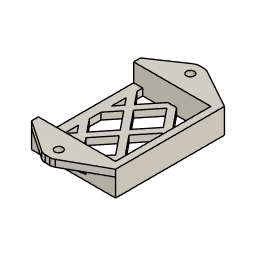
Top Motor Base_ (Autodesk Fusion 360 design; units mm, degrees)
Autodesk Fusion 360 part; units mm, degrees
sketch "Sketch1" plane through (0, 0, 0) normal (0, 0, 1) x (1, 0, 0)
  line L0 (0, 0) -> (-34, 0)
  line L1 (-34, 42) -> (0, 42)
  line L2 (0, 42) -> (0, 0)
  line L3 (-34, -3) -> (-34, 45)
  line L4 (3, -3) -> (-34, -3)
  line L5 (-34, 45) -> (3, 45)
  line L6 (3, 45) -> (3, -3)
  line L7 (-18, 55) -> (-16, 55)
  line L8 (-12, 51) -> (-12, 45)
  line L9 (-12, 45) -> (-22, 45)
  line L10 (-22, 45) -> (-22, 51)
  circle A0 centre (-17, 50) radius 1.75
  arc A1 (-18, 55) -> (-22, 51) centre (-18, 51) ccw
  arc A2 (-12, 51) -> (-16, 55) centre (-16, 51) ccw
  circle A3 centre (-17, -8) radius 1.75
  line L11 (-22, -3) -> (-22, -9)
  arc A4 (-22, -9) -> (-18, -13) centre (-18, -9) ccw
  line L12 (-18, -13) -> (-16, -13)
  arc A5 (-16, -13) -> (-12, -9) centre (-16, -9) ccw
  line L13 (-12, -9) -> (-12, -3)
  line L14 (3, 45) -> (-14.0543, 54.4949)
  line L15 (3, -3) -> (-14.0543, -12.4949)
  line L16 (-34, 45) -> (-20.2422, 54.3125)
  line L17 (-34, -3) -> (-20.2422, -12.3125)
  line L18 (-19.75, -9.5877) -> (-17, -11.1754)
  line L19 (-17, -11.1754) -> (-14.25, -9.5877)
  line L20 (-14.25, -9.5877) -> (-14.25, -6.4123)
  line L21 (-14.25, -6.4123) -> (-17, -4.8246)
  line L22 (-17, -4.8246) -> (-19.75, -6.4123)
  line L23 (-19.75, -6.4123) -> (-19.75, -9.5877)
  point P0 (-22, 55)
  point P1 (-12, 55)
  point P2 (-17, -8)
  dimension "d1" = 34
  dimension "d2" = 42
  dimension "d6" = 10
  dimension "d7" = 10
  dimension "d8" = 3.5
  dimension "d9" = 4
  dimension "d24" = 20
  dimension "d43" = 5
  dimension "d79" = 2.75
  constraint horizontal L0
  constraint vertical L3
  constraint horizontal L1
  constraint vertical L2
  constraint coincident L0.start L2.end
  constraint horizontal L7
  constraint vertical L8
  constraint horizontal L9
  constraint vertical L10
  constraint coincident P0 L7
  constraint coincident P0 L10
  constraint tangent L7 A1
  constraint tangent L10 A1
  constraint coincident P1 L7
  constraint coincident P1 L8
  constraint tangent L7 A2
  constraint tangent L8 A2
  constraint equal A1 A2
  constraint coincident A2 L14.end
  constraint tangent A2 L14
  constraint coincident A5 L15.end
  constraint tangent A5 L15
  constraint coincident L1.start L3
  constraint coincident L0.end L3
  constraint coincident A1 L16.end
  constraint tangent A1 L16
  constraint coincident A4 L17.end
  constraint tangent A4 L17
  constraint coincident P2 A3.centre
  constraint parallel L3 L23
  measures "d1" distance of L0.start L0.end
  measures "d2" distance of L0.start L1.end
  measures "d6" distance of P0 P1
  measures "d7" distance of P0 L9.end
  measures "d8" diameter of A0
  measures "d9" radius of A1
  measures "d24" distance of L6 A0.centre
  measures "d43" distance of L5 A0.centre
  measures "d79" distance of P2 L23
extrude "Extrude1" add sketch "Sketch1" along normal blind 11 contours L0 L1 L2 L3 L4 L5 L6 L9
extrude "Extrude2" add sketch "Sketch1" along normal blind 3 from surface at 8 contours L4 L11 A4 L17 | L4 L11 A4 L12 A5 L13 | L5 L10 A1 L16 | L4 A5 L13 L15 | L5 L7 L8 L9 L10 A1 A2 | L5 L8 A2 L14 | L18 L19 L20 L21 L22 L23
extrude "Extrude5" add sketch "Sketch1" along normal blind 3 contours L0 L1 L2 L3
ref_plane "WorkPlane3" through (0, 21, 0) normal (0, 1, 0) x (0, 0, 1)
sketch "Sketch5" plane through (0, 0, 3) normal (0, 0, 1) x (-1, 0, 0)
  line L0 (30, 0) -> (30, -42)
  line L1 (34, -42) -> (34, 0)
  line L2 (34, 0) -> (0, 0)
  line L3 (0, 0) -> (0, -42)
  line L4 (0, -42) -> (34, -42)
  line L5 (34, -42) -> (34, 0)
  line L6 (0, -21) -> (17, 0)
  line L7 (0, -42) -> (30, -4.9412)
  line L8 (17, -42) -> (30, -25.9412)
  line L9 (17, -42) -> (0, -21)
  line L10 (0, 0) -> (30, -37.0588)
  line L11 (30, -16.0588) -> (17, 0)
  line L12 (18.1659, -41.0562) -> (1.1659, -20.0562)
  line L13 (15.0701, -42) -> (0, -23.384)
  line L14 (1.9299, -42) -> (30, -7.3252)
  line L15 (0, -39.616) -> (30, -2.5572)
  line L16 (18.9299, -42) -> (30, -28.3252)
  line L17 (15.8341, -41.0562) -> (30, -23.5572)
  line L18 (1.1659, -21.9438) -> (18.1659, -0.9438)
  line L19 (0, -18.616) -> (15.0701, 0)
  line L20 (0, -2.384) -> (30, -39.4428)
  line L21 (1.9299, 0) -> (30, -34.6748)
  line L22 (30, -13.6748) -> (18.9299, 0)
  line L23 (30, -18.4428) -> (15.8341, -0.9438)
  dimension "d64" = 42
  dimension "d65" = 4
  dimension "d66" = 1.5
  dimension "d72" = 1.5
  constraint vertical L0
  constraint midpoint L3 L6.start
  constraint midpoint L2 L6.end
  constraint coincident L3.end L4.start
  constraint coincident L0 L7.end
  constraint parallel L6 L7
  constraint midpoint L4 L8.start
  constraint coincident L0 L8.end
  constraint parallel L7 L8
  constraint coincident L2.end L3.start
  constraint coincident L0 L10.end
  constraint parallel L9 L10
  constraint coincident L0 L11.start
  constraint coincident L2 L6.end
  constraint parallel L10 L11
  constraint coincident L6.end L11.end
  constraint coincident L4 L13.start
  constraint coincident L4 L16.start
  constraint coincident L4 L14.start
  constraint coincident L3 L15.start
  constraint coincident L0 L21.end
  constraint coincident L0 L16.end
  constraint coincident L0 L22.start
  constraint coincident L0 L14.end
  constraint coincident L2 L19.end
  constraint coincident L2 L22.end
  constraint coincident L2 L21.start
  constraint coincident L3 L20.start
  constraint coincident L3 L19.start
  constraint coincident L3 L13.end
  constraint coincident L0 L20.end
  constraint coincident L0 L17.end
  constraint coincident L0 L15.end
  constraint coincident L0 L23.start
  measures "d64" distance of L0.start L0.end
  measures "d65" distance of L0 L1
extrude "Extrude6" cut sketch "Sketch5" against normal blind 5 contours L0 L2 L15 L22 | L0 L14 L22 | L0 L4 L16 L20 | L2 L19 L21 | L15 L18 L21 L23 | L0 L14 L17 L21 L23 | L0 L16 L21 | L4 L13 L14 | L3 L19 L20 | L12 L15 L18 L20 | L12 L14 L17 L20 | L3 L13 L15
sketch "Sketch6" plane through (-34, 0, 0) normal (-1, 0, 0) x (0, -1, 0)
  line L0 (-45, 0) -> (3, 0)
  line L1 (3, 0) -> (3, 8)
  line L2 (3, 8) -> (3, 11)
  line L3 (3, 11) -> (0, 11)
  line L4 (0, 11) -> (0, 3)
  line L5 (0, 3) -> (-42, 3)
  line L6 (-42, 3) -> (-42, 11)
  line L7 (-42, 11) -> (-45, 11)
  line L8 (-45, 11) -> (-45, 8)
  line L9 (-45, 8) -> (-45, 0)
  line L10 (3, 8) -> (12.3125, 8)
  line L11 (3, 0) -> (3, 8)
  line L12 (9.5141, 8) -> (3, 2.5254)
  constraint coincident L10 L12.start
  constraint coincident L1 L12.end
extrude "Extrude8" add sketch "Sketch6" against normal blind 3 from surface at -10 contours L1 L10 L11 L12
ref_plane "WorkPlane4" through (-17, 21, 5.5) normal (-1, 0, 0) x (0, -1, 0)
mirror "Mirror4" about plane through (-17, 21, 5.5) normal (-1, 0, 0) of "Extrude8"
mirror "Mirror5" about plane through (0, 21, 0) normal (0, 1, 0) of "Extrude8", "Mirror4"
